Six access compliant mechanism one part-dup (Autodesk Fusion 360 design; units mm, degrees)
Autodesk Fusion 360 part; units mm, degrees
note: some values were not read from the file. Set by a fixed rule: which sketch regions a step uses.
sketch "Sketch1" plane through (0, 0, 0) normal (0, 0, 1) x (1, 0, 0)
  circle A0 centre (0, 0) radius 10
  line L0 (6.3597, 24.6058) -> (-6.3597, 24.6058)
  line L1 (-12.1158, 24.6058) -> (12.1158, 24.6058)
  line L2 (12.1158, 24.6058) -> (12.1158, 30.9361)
  line L3 (12.1158, 30.9361) -> (-12.1158, 30.9361)
  line L4 (-12.1158, 30.9361) -> (-12.1158, 24.6058)
  line L5 (-6.3597, 16.4464) -> (-18.6472, 16.4464) construction
  line L6 (-18.6472, 16.4464) -> (-18.6472, 35.8505) construction
  line L7 (-23.9983, 41.5663) -> (23.9983, 41.5663)
  line L8 (0, -6.1301) -> (0, 107.9633)
  line L9 (-17.1472, 35.8505) -> (-17.1472, 36.8505)
  line L10 (-20.1472, 36.8505) -> (-20.1472, 35.8505)
  line L11 (-6.7685, 16.9464) -> (-17.4085, 16.9464)
  line L12 (-18.1472, 17.6851) -> (-18.1472, 35.6205)
  line L13 (-6.7685, 15.9464) -> (-18.4085, 15.9464)
  line L14 (-19.1472, 16.6851) -> (-19.1472, 35.6205)
  line L15 (-17.9171, 35.8505) -> (-17.1472, 35.8505)
  line L16 (-20.1472, 35.8505) -> (-19.3772, 35.8505)
  arc A1 (-17.9171, 35.8505) -> (-18.1472, 35.6205) centre (-17.9171, 35.6205) ccw
  arc A2 (-19.1472, 35.6205) -> (-19.3772, 35.8505) centre (-19.3772, 35.6205) ccw
  arc A3 (-18.1472, 17.6851) -> (-17.4085, 16.9464) centre (-17.4085, 17.6851) ccw
  arc A4 (-19.1472, 16.6851) -> (-18.4085, 15.9464) centre (-18.4085, 16.6851) ccw
  line L17 (-6.3597, 24.6058) -> (-6.3597, 17.3551)
  line L18 (-6.3597, 15.5376) -> (-6.3597, 7.7171)
  arc A5 (-6.7685, 16.9464) -> (-6.3597, 17.3551) centre (-6.7685, 17.3551) ccw
  arc A6 (-6.3597, 15.5376) -> (-6.7685, 15.9464) centre (-6.7685, 15.5376) ccw
  line L19 (17.1472, 35.8505) -> (17.1472, 36.8505)
  line L20 (20.1472, 36.8505) -> (20.1472, 35.8505)
  line L21 (6.7685, 15.9464) -> (18.4085, 15.9464)
  line L22 (19.1472, 16.6851) -> (19.1472, 35.6205)
  arc A7 (6.7685, 15.9464) -> (6.3597, 15.5376) centre (6.7685, 15.5376) ccw
  arc A8 (18.1472, 35.6205) -> (17.9171, 35.8505) centre (17.9171, 35.6205) ccw
  line L23 (17.9171, 35.8505) -> (17.1472, 35.8505)
  line L24 (18.1472, 17.6851) -> (18.1472, 35.6205)
  line L25 (18.6472, 16.4464) -> (18.6472, 35.8505) construction
  arc A9 (19.3772, 35.8505) -> (19.1472, 35.6205) centre (19.3772, 35.6205) ccw
  arc A10 (17.4085, 16.9464) -> (18.1472, 17.6851) centre (17.4085, 17.6851) ccw
  line L26 (20.1472, 35.8505) -> (19.3772, 35.8505)
  arc A11 (6.3597, 17.3551) -> (6.7685, 16.9464) centre (6.7685, 17.3551) ccw
  arc A12 (18.4085, 15.9464) -> (19.1472, 16.6851) centre (18.4085, 16.6851) ccw
  line L27 (6.7685, 16.9464) -> (17.4085, 16.9464)
  line L28 (6.3597, 16.4464) -> (18.6472, 16.4464) construction
  line L29 (6.3597, 7.7171) -> (6.3597, 15.5376)
  line L30 (6.3597, 17.3551) -> (6.3597, 24.6058)
  line L31 (-20.1472, 36.8505) -> (-26.721, 36.8505)
  line L32 (26.721, 36.8505) -> (20.1472, 36.8505)
  line L33 (17.1472, 36.8505) -> (-17.1472, 36.8505)
  circle A13 centre (-8.4276, 27.7709) radius 1.5
  line L34 (-8.4276, 27.7709) -> (-8.4276, 30.9361) construction
  line L35 (-8.4276, 27.7709) -> (-8.4276, 24.6058) construction
  circle A14 centre (8.4276, 27.7709) radius 1.5
  line L36 (-23.9983, 41.5663) -> (-47.9966, 0)
  line L37 (-47.9966, 0) -> (-23.9983, -41.5663)
  line L38 (-23.9983, -41.5663) -> (23.9983, -41.5663)
  line L39 (23.9983, -41.5663) -> (47.9966, 0)
  line L40 (47.9966, 0) -> (23.9983, 41.5663)
  line L41 (23.9983, 41.5663) -> (-23.9983, 41.5663)
  line L42 (-52.9966, -46.5663) -> (52.9966, -46.5663)
  line L43 (52.9966, -46.5663) -> (52.9966, 46.5663)
  line L44 (52.9966, 46.5663) -> (-52.9966, 46.5663)
  line L45 (-52.9966, 46.5663) -> (-52.9966, -46.5663)
  line L46 (-52.9966, -46.5663) -> (52.9966, 46.5663) construction
  line L47 (52.9966, -46.5663) -> (-52.9966, 46.5663) construction
  circle A15 centre (-44.9358, 38.5055) radius 2
  line L48 (-44.9358, 38.5055) -> (-44.9358, 46.5663) construction
  line L49 (-44.9358, 38.5055) -> (-52.9966, 38.5055) construction
  line L50 (-44.9358, -38.5055) -> (-44.9358, -46.5663) construction
  line L51 (56.4762, -38.5055) -> (52.9966, -38.5055) construction
  line L52 (-18.0602, -2.6115) -> (-23.3802, 6.603)
  line L53 (-24.0233, 8.2394) -> (-40.4218, -1.2283)
  arc A16 (-23.3802, 6.603) -> (-24.3893, 6.8734) centre (-24.02, 6.2336) ccw
  line L54 (-32.8494, -4.9755) -> (-20.7335, -25.9607)
  line L55 (-40.006, -2.4086) -> (-39.6211, -3.0754)
  arc A17 (-10.2761, -13.2765) -> (-10.4257, -13.8348) centre (-10.0718, -13.6305) ccw
  line L56 (-23.5666, 7.9257) -> (-40.3711, -1.7763) construction
  arc A18 (-11.2918, -14.3348) -> (-11.8501, -14.1852) centre (-11.6457, -14.5392) ccw
  line L57 (-47.9966, 0) -> (-23.9983, -41.5663)
  circle A19 centre (-19.8365, -21.184) radius 1.5
  arc A20 (-22.0889, -33.442) -> (-21.7746, -33.5262) centre (-21.8897, -33.3269) ccw
  line L58 (-4.8761, -24.9245) -> (-21.2746, -34.3922)
  line L59 (-6.2421, -24.5585) -> (-21.7746, -33.5262)
  arc A21 (-21.2746, -34.3922) -> (-21.3588, -34.7064) centre (-21.1596, -34.5914) ccw
  line L60 (-23.9983, -41.5663) -> (23.9983, -41.5663)
  line L61 (-20.9739, -35.3732) -> (-21.3588, -34.7064)
  arc A22 (-6.2421, -24.5585) -> (-5.9718, -23.5494) centre (-6.6115, -23.9187) ccw
  line L62 (-24.4891, -6.7952) -> (-18.1293, -17.8106)
  line L63 (-42.4201, -1.2273) -> (-41.1211, -0.4773)
  arc A23 (-4.8761, -24.9245) -> (-4.6057, -23.9154) centre (-5.2455, -24.2847) ccw
  line L64 (-4.9194, -24.3721) -> (-21.7239, -34.0742) construction
  line L65 (-27.3671, -1.8103) -> (-32.8494, -4.9755)
  arc A24 (-18.2098, -3.1699) -> (-18.0602, -2.6115) centre (-18.4142, -2.8159) ccw
  arc A25 (-17.1942, -2.1115) -> (-16.6359, -2.2611) centre (-16.8402, -1.9072) ccw
  line L66 (-17.1942, -2.1115) -> (-23.0142, 7.969)
  arc A26 (-23.0142, 7.969) -> (-24.0233, 8.2394) centre (-23.6539, 7.5996) ccw
  arc A27 (-40.7361, -1.1441) -> (-40.4218, -1.2283) centre (-40.5369, -1.0291) ccw
  arc A28 (-39.9218, -2.0943) -> (-40.006, -2.4086) centre (-39.8068, -2.2935) ccw
  line L67 (-17.4228, -2.7155) -> (-23.5666, 7.9257) construction
  line L68 (-41.1211, -0.4773) -> (-40.7361, -1.1441)
  line L69 (-20.7335, -25.9607) -> (-15.2513, -22.7955)
  circle A29 centre (0, 0) radius 10
  line L70 (-10.4257, -13.8348) -> (-4.6057, -23.9154)
  line L71 (-24.3893, 6.8734) -> (-39.9218, -2.0943)
  line L72 (-11.2918, -14.3348) -> (-5.9718, -23.5494)
  line L73 (-9.8631, 1.6491) -> (-16.6359, -2.2611)
  line L74 (-10.2761, -13.2765) -> (-3.5034, -9.3662)
  circle A30 centre (-28.2641, -6.5869) radius 1.5
  line L75 (-22.2729, -36.1232) -> (-20.9739, -35.3732)
  line L76 (-39.6211, -3.0754) -> (-40.9201, -3.8254)
  line L77 (-22.4739, -32.7752) -> (-23.7729, -33.5252)
  line L78 (-45.5627, 4.2158) -> (-42.4201, -1.2273)
  line L79 (-40.9201, -3.8254) -> (-23.7729, -33.5252)
  line L80 (-23.9983, -41.5663) -> (-47.9966, 0)
  line L81 (-22.2729, -36.1232) -> (-19.1304, -41.5663)
  line L82 (-19.8365, -21.184) -> (-17.0954, -19.6014) construction
  line L83 (-15.2513, -22.7955) -> (-27.3671, -1.8103)
  line L84 (-18.1293, -17.8106) -> (-11.8501, -14.1852)
  line L85 (-19.8365, -21.184) -> (-22.5776, -22.7666) construction
  line L86 (-18.2098, -3.1699) -> (-24.4891, -6.7952)
  line L87 (-22.0889, -33.442) -> (-22.4739, -32.7752)
  line L88 (-11.0631, -13.7309) -> (-4.9194, -24.3721) construction
  line L89 (-23.9983, 41.5663) -> (-47.9966, 0)
  line L90 (11.2918, -14.3348) -> (5.9718, -23.5494)
  line L91 (4.8761, -24.9245) -> (21.2746, -34.3922)
  arc A31 (5.9718, -23.5494) -> (6.2421, -24.5585) centre (6.6115, -23.9187) ccw
  line L92 (20.7335, -25.9607) -> (32.8494, -4.9755)
  line L93 (22.0889, -33.442) -> (22.4739, -32.7752)
  arc A32 (16.6359, -2.2611) -> (17.1942, -2.1115) centre (16.8402, -1.9072) ccw
  line L94 (4.9194, -24.3721) -> (21.7239, -34.0742) construction
  arc A33 (18.0602, -2.6115) -> (18.2098, -3.1699) centre (18.4142, -2.8159) ccw
  line L95 (23.9983, -41.5663) -> (47.9966, 0)
  circle A34 centre (28.2641, -6.5869) radius 1.5
  arc A35 (40.006, -2.4086) -> (39.9218, -2.0943) centre (39.8068, -2.2935) ccw
  line L96 (24.0233, 8.2394) -> (40.4218, -1.2283)
  line L97 (24.3893, 6.8734) -> (39.9218, -2.0943)
  arc A36 (40.4218, -1.2283) -> (40.7361, -1.1441) centre (40.5369, -1.0291) ccw
  line L98 (47.9966, 0) -> (23.9983, 41.5663)
  line L99 (41.1211, -0.4773) -> (40.7361, -1.1441)
  arc A37 (24.3893, 6.8734) -> (23.3802, 6.603) centre (24.02, 6.2336) ccw
  line L100 (18.1293, -17.8106) -> (24.4891, -6.7952)
  line L101 (22.2729, -36.1232) -> (20.9739, -35.3732)
  arc A38 (24.0233, 8.2394) -> (23.0142, 7.969) centre (23.6539, 7.5996) ccw
  line L102 (23.5666, 7.9257) -> (40.3711, -1.7763) construction
  line L103 (15.2513, -22.7955) -> (20.7335, -25.9607)
  arc A39 (11.8501, -14.1852) -> (11.2918, -14.3348) centre (11.6457, -14.5392) ccw
  arc A40 (10.4257, -13.8348) -> (10.2761, -13.2765) centre (10.0718, -13.6305) ccw
  line L104 (10.4257, -13.8348) -> (4.6057, -23.9154)
  arc A41 (4.6057, -23.9154) -> (4.8761, -24.9245) centre (5.2455, -24.2847) ccw
  arc A42 (21.3588, -34.7064) -> (21.2746, -34.3922) centre (21.1596, -34.5914) ccw
  arc A43 (21.7746, -33.5262) -> (22.0889, -33.442) centre (21.8897, -33.3269) ccw
  line L105 (11.0631, -13.7309) -> (4.9194, -24.3721) construction
  line L106 (20.9739, -35.3732) -> (21.3588, -34.7064)
  line L107 (32.8494, -4.9755) -> (27.3671, -1.8103)
  circle A44 centre (0, 0) radius 10
  line L108 (17.1942, -2.1115) -> (23.0142, 7.969)
  line L109 (6.2421, -24.5585) -> (21.7746, -33.5262)
  line L110 (18.0602, -2.6115) -> (23.3802, 6.603)
  line L111 (3.5034, -9.3662) -> (10.2761, -13.2765)
  line L112 (16.6359, -2.2611) -> (9.8631, 1.6491)
  circle A45 centre (19.8365, -21.184) radius 1.5
  line L113 (42.4201, -1.2273) -> (41.1211, -0.4773)
  line L114 (22.4739, -32.7752) -> (23.7729, -33.5252)
  line L115 (39.6211, -3.0754) -> (40.9201, -3.8254)
  line L116 (19.1304, -41.5663) -> (22.2729, -36.1232)
  line L117 (23.7729, -33.5252) -> (40.9201, -3.8254)
  line L118 (47.9966, 0) -> (23.9983, -41.5663)
  line L119 (42.4201, -1.2273) -> (45.5627, 4.2158)
  line L120 (28.2641, -6.5869) -> (25.523, -5.0043) construction
  line L121 (27.3671, -1.8103) -> (15.2513, -22.7955)
  line L122 (24.4891, -6.7952) -> (18.2098, -3.1699)
  line L123 (28.2641, -6.5869) -> (31.0053, -8.1695) construction
  line L124 (11.8501, -14.1852) -> (18.1293, -17.8106)
  line L125 (40.006, -2.4086) -> (39.6211, -3.0754)
  line L126 (17.4228, -2.7155) -> (23.5666, 7.9257) construction
  line L127 (-23.9983, -41.5663) -> (23.9983, -41.5663)
  line L128 (-74.0845, 0) -> (69.1863, 0) construction
  circle A46 centre (44.9358, 38.5055) radius 2
  circle A47 centre (44.9358, -38.5055) radius 2
  circle A48 centre (-44.9358, -38.5055) radius 2
  point P0 (0, 24.6058)
  point P1 (0, 41.5663)
  point P2 (12.1158, 30.9361)
  point P3 (12.1158, 24.6058)
  point P4 (6.3597, 24.6058)
  point P5 (-35.9975, -20.7832)
  point P6 (-27.3671, -1.8103)
  point P7 (-21.3092, -12.3029)
  point P8 (-32.8494, -4.9755)
  point P9 (-24.4891, -6.7952)
  point P10 (35.9975, -20.7832)
  point P11 (15.2513, -22.7955)
  point P12 (21.3092, -12.3029)
  point P13 (20.7335, -25.9607)
  point P14 (18.1293, -17.8106)
  dimension "d1" = 20
  dimension "d2" = 16.8886
  dimension "d3" = 24.2316
  dimension "d4" = 6.3304
  dimension "d5" = 1
  dimension "d6" = 3
  dimension "d9" = 0.23
  dimension "d10" = 0.7387
  dimension "d11" = 0.4087
  dimension "d12" = 3
  dimension "d13" = 5
  dimension "d14" = 5
  dimension "d15" = 4
  constraint coincident A0.centre A29.centre
  constraint vertical L29
  constraint horizontal L0
  constraint coincident A0 L18.end
  constraint coincident A0 L29.start
  constraint horizontal L1
  constraint vertical L2
  constraint horizontal L3
  constraint vertical L4
  constraint midpoint L0 P0
  constraint midpoint L1 P0
  constraint perpendicular L5 L6
  constraint horizontal L7
  constraint horizontal L32
  constraint vertical L8
  constraint coincident L8 P1
  constraint coincident A0.centre L8
  constraint vertical L9
  constraint vertical L10
  constraint coincident L10.start L32
  constraint horizontal L15
  constraint horizontal L16
  constraint tangent L15 A1
  constraint tangent L12 A1
  constraint tangent L14 A2
  constraint tangent L16 A2
  constraint equal A1 A2
  constraint tangent L11 A3
  constraint tangent L12 A3
  constraint tangent L13 A4
  constraint tangent L14 A4
  constraint equal A3 A4
  constraint vertical L17
  constraint vertical L18
  constraint tangent L11 A5
  constraint tangent L17 A5
  constraint tangent L13 A6
  constraint tangent L18 A6
  constraint equal A5 A6
  constraint symmetric L0.end L8 P4
  constraint symmetric L1.start L8 P3
  constraint symmetric L3.end L8 P2
  constraint symmetric L5.start L8 L28.start
  constraint symmetric L5.end L8 L25.start
  constraint symmetric L6.end L8 L25.end
  constraint symmetric L8 L10.end L20.end
  constraint symmetric L8 L9.start L19.start
  constraint symmetric L8 L9.end L19.end
  constraint symmetric L8 L10.start L20.start
  constraint symmetric L8 L15.start A8.end
  constraint symmetric L8 L12.end A8.start
  constraint symmetric L8 A1 A8
  constraint symmetric L8 L14.end L22.end
  constraint symmetric L8 L16.end A9.start
  constraint symmetric L8 A2 A9
  constraint symmetric L8 L11.end A10.start
  constraint symmetric L8 L12.start L24.start
  constraint symmetric L8 A3 A10
  constraint symmetric L8 L13.end L21.end
  constraint symmetric L8 L14.start L22.start
  constraint symmetric L8 A4 A12
  constraint symmetric L8 L11.start A11.end
  constraint symmetric L8 L17.end A11.start
  constraint symmetric L8 A5 A11
  constraint symmetric L8 L13.start L21.start
  constraint symmetric L8 L18.start A7.end
  constraint symmetric L8 A6 A7
  constraint collinear L31 L32
  constraint collinear L32 L33
  constraint coincident A13.centre L34.start
  constraint coincident L3 L34.end
  constraint perpendicular L3 L34
  constraint coincident L1 L35.end
  constraint perpendicular L1 L35
  constraint equal L34 L35
  constraint symmetric L8 A13 A14
  constraint horizontal L41
  constraint coincident L7 P1
  constraint coincident L40 L32.start
  constraint coincident L36 L31.end
  constraint horizontal L42
  constraint perpendicular L42 L43
  constraint parallel L42 L44
  constraint parallel L43 L45
  constraint coincident L46 A0.centre
  constraint coincident L47 A0.centre
  constraint coincident A15.centre L48.start
  constraint coincident L44 L48.end
  constraint perpendicular L44 L48
  constraint coincident L45 L49.end
  constraint perpendicular L45 L49
  constraint equal L48 L49
  constraint coincident L42 L50.end
  constraint perpendicular L42 L50
  constraint equal L48 L50
  constraint coincident L43 L51.end
  constraint perpendicular L43 L51
  constraint perpendicular L43 L128
  constraint symmetric L8 A15 A46
  constraint symmetric A15 L128 A48
  constraint symmetric L128 A46 A47
  measures "d1" diameter of A0
  measures "d2" distance of L29.start L0.start
  measures "d3" distance of L1.start P3
  measures "d4" distance of P3 P2
  measures "d5" distance of L10.end L10.start
  measures "d6" distance of L10.end L9.start
  measures "d9" radius of A1
  measures "d10" radius of A3
  measures "d11" radius of A5
  measures "d12" diameter of A13
  measures "d13" distance of L41 L44
  measures "d14" distance of L36.end L45
  measures "d15" diameter of A15
extrude "Extrude1" add sketch "Sketch1" along normal blind 1.5 contours A0 A29 A44 | A0 L38 L39 L40 L60 A29 L91 A32 L95 L96 A36 L98 L99 L101 A38 A40 L104 A41 A42 L106 A44 L108 L111 L112 L113 L116 L118 L119 L127 | A0 L0 L1 L7 L8 L19 L20 L21 L22 A7 A8 L23 L24 A9 A10 L26 A11 A12 L27 L29 L30 L32 L33 L40 L41 A29 L98 A44 | A0 L36 L37 L38 L53 A17 L57 L58 A21 L60 L61 L63 A23 A25 L66 A26 A27 L68 A29 L70 L73 L74 L75 L78 L80 L81 L89 A44 L127 | A0 L0 L1 L7 L8 L9 L10 L11 L12 L13 L14 L15 L16 A1 A2 A3 A4 L17 L18 A5 A6 L31 L33 L36 L41 A29 L89 A44 | L0 L1 L2 L3 L8 | L0 L1 L3 L4 L8 | L42 L43 L44 L45 | L54 L62 L65 L69 L83 | L92 L100 L103 L107 L121
extrude "Extrude2" add sketch "Sketch1" along normal blind 0.5 contours A13 | A14 | A19 | A30 | A34 | A45
